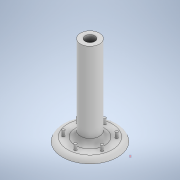
# Autodesk Inventor part: flume-nursery
Saved by Autodesk Inventor 2021 (Build 250183000, 183)
## iProperties
Created: 2020-08-01
Part Number: flume-nursery
Material: Generic
Document SubType Name: Modeling
Designer: Scratch
Density: 1 g/cm^3
Appearance: Default
Author: Scratch
Autodesk Inventor part; units mm, degrees
ref_plane "YZ Plane" through (0, 0, 0) normal (1, 0, 0) x (0, 1, 0)
ref_plane "XZ Plane" through (0, 0, 0) normal (0, 1, 0) x (-1, 0, 0)
ref_plane "XY Plane" through (0, 0, 0) normal (0, 0, 1) x (1, 0, 0)
sketch "Sketch1" plane through (0, 0, 0) normal (0, 0, 1) x (1, 0, 0)
  line L0 (1.1948, 21.5189) -> (2.2959, 21.5189)
  line L1 (6.6309, 0) -> (1.1948, 0)
  line L2 (1.1948, 0.9728) -> (1.1948, 21.5189)
  line L3 (2.2959, 21.5189) -> (2.2959, 0.9728)
  line L4 (2.2959, 0.9728) -> (6.6309, 0.9728)
  line L5 (6.6309, 0.9728) -> (6.6309, 0)
  line L6 (1.1948, 0.9728) -> (0, 0.9728)
  line L7 (0, 0.9728) -> (0, 0)
  line L8 (0, 0) -> (1.1948, 0)
  constraints: 18 end point, 2 horizontal, 2 perpendicular, 2 point on line, 1 parallel, 1 vertical
revolve "Revolution1" add sketch "Sketch1" angle 360 about axis through (0, 0.9728, 0) along (0, -1, 0)
fillet "Fillet1" radius 1.27 1 edges at (-2.2959, 0.9728, 0)
fillet "Fillet2" radius 1.27 1 edges at (-6.6309, 0.9728, 0)
sketch "Sketch2" plane through (0, 0.9728, 0) normal (0, 1, 0) x (1, 0, 0)
  circle A0 centre (0, 0) radius 3.5659 projected
  circle A1 centre (0, 0) radius 5.3961 projected
  circle A2 centre (-0.0164, -4.5633) radius 0.3175
  circle A3 centre (1.841, -4.1755) radius 0.3175
  circle A4 centre (3.3802, -3.0657) radius 0.3175
  circle A5 centre (4.3349, -1.4258) radius 0.3175
  circle A6 centre (4.54, 0.4606) radius 0.3175
  circle A7 centre (3.9602, 2.2674) radius 0.3175
  circle A8 centre (2.6955, 3.6821) radius 0.3175
  circle A9 centre (0.9648, 4.4602) radius 0.3175
  circle A10 centre (-0.9327, 4.467) radius 0.3175
  circle A11 centre (-2.6689, 3.7015) radius 0.3175
  circle A12 centre (-3.9437, 2.2959) radius 0.3175
  circle A13 centre (-4.5366, 0.4933) radius 0.3175
  circle A14 centre (-4.345, -1.3945) radius 0.3175
  circle A15 centre (-3.4022, -3.0412) radius 0.3175
  circle A16 centre (-1.8711, -4.1621) radius 0.3175
  point P0 (0, 0)
  dimension "d3" = 0.635
  dimension "d6" = 360
  constraints: 15 centre point, 31 other
  measures "d3" diameter of A2
extrude "Extrusion1" add sketch "Sketch2" along normal blind 1.27 contours A15
pattern_circular "Circular Pattern1" count 6 over 360 about axis through (0, -10, 0) along (0, 1, 0) of "Extrusion1"
body "Solid1"
